# Autodesk Inventor part: Roller Chain Sprocket1
Saved by Autodesk Inventor 2016 (Build 200138000, 138)
## iProperties
Created: 2016-04-25
Part Number: Roller Chain Sprocket1
Material: Steel
Document SubType Name: Modeling
Designer: Henrik Samuelsson
Density: 1 g/cm^3
Appearance: Steel
CustomPartVersion: 1
Author: Henrik Samuelsson
Autodesk Inventor part; units mm, degrees
ref_plane "YZ Plane" through (0, 0, 0) normal (1, 0, 0) x (0, 1, 0)
ref_plane "XZ Plane" through (0, 0, 0) normal (0, 1, 0) x (-1, 0, 0)
sketch "Theoretical Tooth Profile" plane through (0, 0, 0) normal (0, 0, 1) x (1, 0, 0)
  circle A0 centre (0, 0) radius 88.7332 construction
  line L0 (0, 0) -> (0, 88.7332) construction
  line L1 (0, 0) -> (28.8116, 83.9254) construction
  circle A1 centre (0, 0) radius 93.3052
  arc A2 (-4.5387, 85.167) -> (4.5387, 85.167) centre (0, 88.7332) ccw
  line L2 (0, 88.7332) -> (28.8116, 83.9254) construction
  line L3 (0, 88.7332) -> (7.19, 94.3826) construction
  line L4 (7.19, 94.3826) -> (-6.5296, 88.5292) construction
  arc A3 (9.154, 92.855) -> (7.0777, 89.8137) centre (15.7838, 86.0993) ccw
  arc A4 (-7.0777, 89.8137) -> (-9.154, 92.855) centre (-15.7838, 86.0993) ccw
  line L5 (-15.7838, 86.0993) -> (-7.0777, 89.8137) construction
  arc A5 (-6.5296, 88.5292) -> (-4.5387, 85.167) centre (7.19, 94.3826) ccw
  line L6 (-6.5296, 88.5292) -> (-7.0777, 89.8137)
  arc A6 (4.5387, 85.167) -> (6.5296, 88.5292) centre (-7.19, 94.3826) ccw
  line L7 (7.0777, 89.8137) -> (6.5296, 88.5292)
  line L8 (0, 0) -> (15.3575, 92.0326) construction
  point P0 (14.4058, 86.3293)
  dimension "d0" = 177.4663
  dimension "d2" = 18.947
  dimension "d3" = 5.7721
  dimension "d10" = 128.158
  dimension "d11" = 15.053
  dimension "d12" = 9.144
  dimension "d13" = 14.9162
  dimension "d14" = 16.002
  dimension "d23" = 5.7822
  constraints: 18 end point, 15 point on circle, 7 centre point, 3 coincident, 3 point on line, 3 symmetric about line, 3 tangent, 1 equal radius, 1 midpoint, 1 parallel, 1 vertical, 1 other
  measures "d0" diameter of A0
  measures "d2" angle of L1 L0
  measures "d3" radius of A2
  measures "d10" angle of L3 L0
  measures "d11" angle of L4 L3
  measures "d12" distance of L2.start L3.end
  measures "d13" distance of L3.end L4.end
  measures "d14" distance of A3.centre L0.end
  measures "d23" distance from line of L8.end L2
sketch "Tooth Profile" plane through (0, 0, 0) normal (0, 0, 1) x (1, 0, 0)
  circle A0 centre (0, 0) radius 93.3052 projected
  line L0 (0, 0) -> (0, 88.7332) construction
  line L1 (0, 88.7332) -> (5.3378, 86.5365) construction
  arc A1 (-5.3378, 86.5365) -> (5.3378, 86.5365) centre (0, 88.7332) ccw
  line L2 (-5.3378, 86.5365) -> (0, 88.7332) construction
  arc A2 (-5.3378, 86.5365) -> (-8.945, 92.8754) centre (-31.9741, 75.575) ccw
  arc A3 (8.945, 92.8754) -> (5.3378, 86.5365) centre (31.9741, 75.575) ccw
  dimension "d44" = 135.263
  dimension "d45" = 5.7721
  dimension "d46" = 28.8036
  constraints: 8 point on circle, 7 end point, 3 centre point, 2 tangent, 1 coincident, 1 equal radius, 1 symmetric about line, 1 vertical
  measures "d44" angle of L1 L2
  measures "d45" radius of A1
  measures "d46" radius of A3
sketch "Section Profile" plane through (0, 0, 0) normal (1, 0, 0) x (0, 1, 0)
  line L0 (93.3052, 0) -> (-93.3052, 0) projected
  line L1 (75.433, 7.4636) -> (-75.433, 7.4636)
  line L2 (-75.433, 7.4636) -> (-75.433, -7.4636)
  line L3 (-75.433, -7.4636) -> (75.433, -7.4636)
  line L4 (75.433, -7.4636) -> (75.433, 7.4636)
  line L5 (75.433, 7.4636) -> (93.3052, 7.4636) construction
  line L6 (93.3052, 7.4636) -> (93.3052, -7.4636) construction
  line L7 (93.3052, -7.4636) -> (75.433, -7.4636) construction
  line L8 (75.433, -7.4636) -> (75.433, 7.4636)
  arc A0 (93.3052, 4.6274) -> (83.3225, 7.4636) centre (83.3225, -11.5229) ccw
  arc A1 (83.3225, -7.4636) -> (93.3052, -4.6274) centre (83.3225, 11.5229) ccw
  line L9 (83.3225, 7.4636) -> (0, 7.4636)
  line L10 (0, 7.4636) -> (0, -7.4636)
  line L11 (0, -7.4636) -> (83.3225, -7.4636)
  line L12 (0, 7.4636) -> (0, -7.4636)
  line L13 (93.3052, 4.6274) -> (93.3052, -4.6274)
  point P0 (0, 0)
  point P1 (0, 0)
  dimension "d30" = 14.9272
  dimension "d31" = 150.8659
  dimension "d32" = 14.9272
  dimension "d33" = 2.8362
  dimension "d34" = 18.9865
  dimension "d43" = 7.4636
  constraints: 26 end point, 7 midpoint, 5 perpendicular, 4 parallel, 4 point on circle, 3 point on line, 3 symmetric about line, 2 centre point, 2 horizontal, 2 tangent, 1 collinear, 1 other
  measures "d30" distance between parallel lines of L7 L5
  measures "d31" distance between parallel lines of L2 L4
  measures "d32" distance between parallel lines of L3 L1
  measures "d33" distance from line of L13.start L5
  measures "d34" radius of A0
  measures "d43" distance between parallel lines of L3 L0
revolve "Shroud" add sketch "Section Profile" angle 360 about axis through (0, 0, 7.4636) along (0, 0, -1) contours L10 L3 L2 L0 | L0 L2 L1 L10
revolve "Strand" add sketch "Section Profile" angle 360 about axis through (0, 0, 7.4636) along (0, 0, -1) contours L13 A1 L11 L4 L0 | L0 L4 L9 A0 L13 | L4 L3 L10 L0 | L0 L10 L1 L4
pattern_of_one "Strand Pattern"
extrude "Theoretical Tooth" cut sketch "Theoretical Tooth Profile" along normal through all both and the other way through all contours A3 L7 A6 A2 A5 L6 A4 A1 picked at (0, 89.8238)
extrude "Tooth" [suppressed]
pattern_circular "Tooth Pattern" count 19 over 360 about axis through (0, 0, -10) along (0, 0, 1) of "Theoretical Tooth"
ref_plane "Timing Plane" through (0, 88.7332, 0) normal (1, 0, 0) x (0, 1, 0)
equation "\"d3\" = 0.5 * da_Dr + da_SC"
equation "\"d12\" = 0.8 * da_Dr"
equation "\"d13\" = 1.3 * da_Dr + da_SC"
equation "\"d14\" = 1.4 * da_Dr"
equation "\"d23\" = da_Ha"
equation "\"d44\" = da_Alfa"
equation "\"d45\" = da_Ri"
equation "\"d46\" = da_Re"
equation "\"d30\" = da_Bf"
equation "\"d31\" = da_Ds"
equation "\"d32\" = da_Bs"
equation "\"d33\" = da_Ba"
equation "\"d34\" = da_Rx"
equation "\"d40\" = da_pt"
equation "\"form_type\" = 0"
equation "\"da_p\" = 29.21"
equation "\"da_Dr\" = 11.43"
equation "\"da_SC\" = 0.05715"
equation "\"da_Ha\" = 5.7822"
equation "\"da_pt\" = 25"
equation "\"da_Bf\" = 14.9272"
equation "\"da_Ba\" = 2.83617"
equation "\"da_Rx\" = 18.9865"
equation "\"da_Ra\" = 1.27"
equation "\"da_Bs\" = 14.9272"
equation "\"da_Ds\" = 150.86593"
equation "\"da_Re\" = 28.8036"
equation "\"da_Ri\" = 5.77215"
equation "\"da_Alfa\" = 135.263deg"
body "Solid1"
